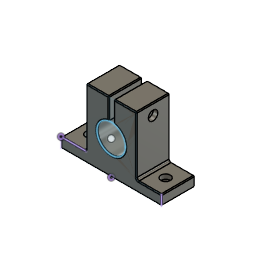
Support Block (Autodesk Fusion 360 design; units mm, degrees)
part number: 2026-05-14-16-39-01-021
Autodesk Fusion 360 part; units mm, degrees
sketch "Sketch1" plane through (0, 0, 0) normal (0, 1, 0) x (1, 0, 0)
  line L0 (-31.75, 12.7) -> (31.75, 12.7)
  line L1 (38.1, 6.35) -> (38.1, -6.35)
  line L2 (31.75, -12.7) -> (-31.75, -12.7)
  line L3 (-38.1, -6.35) -> (-38.1, 6.35)
  line L4 (38.1, -6.35) -> (38.1, -12.7)
  line L5 (38.1, -12.7) -> (31.75, -12.7)
  line L6 (38.1, 6.35) -> (38.1, 12.7)
  line L7 (38.1, 12.7) -> (31.75, 12.7)
  line L8 (-38.1, 6.35) -> (-38.1, 12.7)
  line L9 (-38.1, 12.7) -> (-31.75, 12.7)
  line L10 (-38.1, -6.35) -> (-38.1, -12.7)
  line L11 (-38.1, -12.7) -> (-31.75, -12.7)
  point P0 (-38.1, 12.7)
  point P1 (38.1, 12.7)
  point P2 (38.1, -12.7)
  point P3 (-38.1, -12.7)
  constraint horizontal L0
  constraint vertical L1
  constraint horizontal L2
  constraint vertical L3
  constraint coincident P0 L0
  constraint coincident P0 L3
  constraint coincident P3 L2
  constraint coincident P3 L3
  constraint coincident P1 L0
  constraint coincident P1 L1
  constraint coincident P2 L1
  constraint coincident P2 L2
  constraint coincident P2 L4.end
  constraint coincident P1 L6.end
  constraint coincident P0 L8.end
  constraint coincident P3 L10.end
extrude "Extrude1" add sketch "Sketch1" along normal blind 7.62
sketch "Sketch2" plane through (0, 7.62, 0) normal (0, 1, 0) x (-1, 0, 0)
  line L0 (38.1, -12.7) -> (38.1, 12.7)
  line L1 (38.1, 12.7) -> (-38.1, 12.7)
  line L2 (-38.1, 12.7) -> (-38.1, -12.7)
  line L3 (-38.1, -12.7) -> (38.1, -12.7)
  line L4 (-19.05, 12.7) -> (19.05, 12.7)
  line L5 (19.05, 12.7) -> (19.05, -12.7)
  line L6 (19.05, -12.7) -> (-19.05, -12.7)
  line L7 (-19.05, -12.7) -> (-19.05, 12.7)
  line L8 (-19.05, 12.7) -> (19.05, -12.7) construction
  line L9 (19.05, 12.7) -> (-19.05, -12.7) construction
  dimension "d12" = 38.1
  constraint horizontal L4
  constraint perpendicular L4 L5
  constraint parallel L4 L6
  constraint parallel L5 L7
  constraint coincident L8 origin
  constraint coincident L9 origin
  constraint coincident L1 L4.start
  measures "d12" distance of L5 L7
extrude "Extrude2" add sketch "Sketch2" along normal blind 44.45 contours L1 L3 L4 L5 L6 L7
sketch "Sketch3" plane through (0, 0, 12.7) normal (0, 0, 1) x (1, 0, 0)
  line L0 (-38.1, 0) -> (38.1, 0)
  line L1 (38.1, 7.62) -> (19.05, 7.62)
  line L2 (19.05, 7.62) -> (19.05, 52.07)
  line L3 (19.05, 52.07) -> (-19.05, 52.07)
  line L4 (-19.05, 52.07) -> (-19.05, 7.62)
  circle A0 centre (0, 25.4) radius 10.8585
  line L5 (38.1, 0) -> (38.1, 7.62)
  line L6 (-19.05, 7.62) -> (-38.1, 7.62)
  line L7 (-38.1, 7.62) -> (-38.1, 0)
  dimension "d15" = 25.4
  dimension "d16" = 21.717
  dimension "d47" = 25.4
  measures "d15" distance of origin A0.centre
  measures "d16" diameter of A0
  measures "d47" distance of origin A0.centre
extrude "Extrude3" cut sketch "Sketch3" against normal blind 25.4 contours A0
sketch "Sketch4" plane through (0, 52.07, 0) normal (0, 1, 0) x (-1, 0, 0)
  line L0 (-19.05, -12.7) -> (19.05, -12.7)
  line L1 (19.05, -12.7) -> (19.05, 12.7)
  line L2 (19.05, 12.7) -> (-19.05, 12.7)
  line L3 (-19.05, 12.7) -> (-19.05, -12.7)
  line L4 (-1.905, -12.7) -> (1.905, -12.7)
  line L5 (1.905, -12.7) -> (1.905, 12.7)
  line L6 (1.905, 12.7) -> (-1.905, 12.7)
  line L7 (-1.905, 12.7) -> (-1.905, -12.7)
  line L8 (-1.905, -12.7) -> (1.905, 12.7) construction
  line L9 (1.905, -12.7) -> (-1.905, 12.7) construction
  dimension "d19" = 3.81
  constraint horizontal L4
  constraint perpendicular L4 L5
  constraint parallel L4 L6
  constraint parallel L5 L7
  constraint coincident L8 origin
  constraint coincident L9 origin
  constraint coincident L0 L4.start
  measures "d19" distance of L5 L7
extrude "Extrude4" cut sketch "Sketch4" along normal up to surface contours L0 L2 L4 L5 L6 L7 end surface at (10.8045, 24.3188, -4.2333)
fillet "Fillet1" radius 1.524 1 edges at (19.05, 7.62, 0)
fillet "Fillet1" radius 1.524 1 edges at (-19.05, 7.62, 0)
chamfer "Chamfer1" distance 0.635 angle 45 34 edges at (-19.05, 30.607, -12.7) (-19.05, 30.607, 12.7) (-19.4964, 8.0664, 12.7) (-29.337, 7.62, 12.7) (-19.4964, 8.0664, -12.7) (-29.337, 7.62, -12.7) (19.4964, 8.0664, -12.7) (29.337, 7.62, -12.7) (19.05, 30.607, -12.7) (29.337, 7.62, 12.7) (19.4964, 8.0664, 12.7) (19.05, 30.607, 12.7) (0, 0, -12.7) (-38.1, 0, 0) (-38.1, 3.81, -12.7) (38.1, 3.81, -12.7) (38.1, 0, 0) (38.1, 7.62, 0) (-38.1, 7.62, 0) (38.1, 3.81, 12.7) (0, 0, 12.7) (-38.1, 3.81, 12.7) (1.905, 44.08, -12.7) (1.905, 44.08, 12.7) (-1.905, 52.07, 0) (-1.905, 44.08, 12.7) (-1.905, 44.08, -12.7) (-10.4775, 52.07, -12.7) (-19.05, 52.07, 0) (-10.4775, 52.07, 12.7) (10.4775, 52.07, -12.7) (1.905, 52.07, 0) (19.05, 52.07, 0) (10.4775, 52.07, 12.7)
chamfer "Chamfer3" distance 0.762 angle 45 2 edges at (0, 14.5415, -12.7) (0, 14.5415, 12.7)
ref_plane "WorkPlane1" through (0, 26.035, 0) normal (0, 0, -1) x (-1, 0, 0)
sketch "Sketch5" plane through (0, 7.62, 0) normal (0, 1, 0) x (-1, 0, 0)
  line L0 (37.465, 12.065) -> (20.574, 12.065)
  line L1 (20.574, 12.065) -> (20.574, -12.065)
  line L2 (20.574, -12.065) -> (37.465, -12.065)
  line L3 (37.465, -12.065) -> (37.465, 12.065)
  line L4 (38.1, -12.065) -> (38.1, 12.065)
  line L5 (-38.1, 12.065) -> (-38.1, -12.065)
  point P0 (28.575, 0)
  point P1 (-28.575, 0)
  dimension "d33" = 9.525
  dimension "d34" = 9.525
  measures "d33" distance of P0 L4
  measures "d34" distance of P1 L5
hole "Hole1" at (-28.575, 7.62, 0) at (28.575, 7.62, 0) direction (0, -1, 0) diameter 3.6576 end through all counterbore diameter 7.1374 counterbore depth 3.5052
hole "Hole2" at (19.05, 43.7629, 0) direction (-1, 0, 0) diameter 2.7686 depth 33.02 tip angle 118 counterbore diameter 7.1374 counterbore depth 3.5052
thread "Thread1" "ANSI Unified Screw Threads 0.138(#6) 6-32 UNC 6-32 UNC 3B" thread offset 0 thread depth 5.9436
move_body "Move1" bodies 1 to x (1, 0, 0) y (0, 1, 0) z (0, 0, 1) at (-152.4, 0, 0)
move_body "Move2" bodies 1 to x (1, 0, 0) y (0, 1, 0) z (0, 0, 1) at (152.4, 0, 0)
